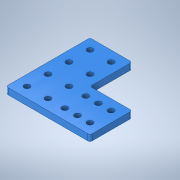
# Autodesk Inventor part: 90deg_4040Bracket
Saved by Autodesk Inventor 2021 (Build 250183000, 183)
## iProperties
Created: 2021-02-03
Part Number: 90deg_4040Bracket
Material: Generic
Document SubType Name: Modeling
Designer: Jorian Brusind
Density: 1 g/cm^3
Appearance: Cyan
Author: Jorian Brusind
Autodesk Inventor part; units mm, degrees
ref_plane "YZ Plane" through (0, 0, 0) normal (1, 0, 0) x (0, 1, 0)
ref_plane "XZ Plane" through (0, 0, 0) normal (0, 1, 0) x (-1, 0, 0)
ref_plane "XY Plane" through (0, 0, 0) normal (0, 0, 1) x (1, 0, 0)
sketch "Sketch1" plane through (0, 0, 0) normal (0, 1, 0) x (-1, 0, 0)
  line L0 (0, 0) -> (40, 0)
  line L1 (40, 0) -> (40, -40)
  line L2 (40, -40) -> (0, -40)
  line L3 (0, -40) -> (0, 0)
  line L4 (40, 0) -> (80, 0)
  line L5 (80, 0) -> (80, -80)
  line L6 (80, -80) -> (40, -80)
  line L7 (40, -80) -> (40, 0)
  dimension "d0" = 40
  dimension "d1" = 40
  dimension "d2" = 40
  dimension "d3" = 80
  constraints: 16 end point, 4 parallel, 2 horizontal, 2 perpendicular
  measures "d0" distance of L1.end L2.end
  measures "d1" distance of L0.end L1.end
  measures "d2" distance of L5.end L6.end
  measures "d3" distance of L4.end L5.end
extrude "Extrusion1" add sketch "Sketch1" along normal blind 6
sketch "Sketch2" plane through (0, 6, 0) normal (0, 1, 0) x (1, 0, 0)
  line L0 (0, 0) -> (0, 40) projected
  line L1 (0, 0) -> (0, 10)
  line L2 (0, 40) -> (0, 30)
  circle A0 centre (-10, 10) radius 2.75
  line L3 (-80, 0) -> (0, 0) projected
  circle A1 centre (-22, 10) radius 2.75
  circle A2 centre (-34, 10) radius 2.75
  circle A3 centre (-10, 30) radius 2.75
  circle A4 centre (-22, 30) radius 2.75
  circle A5 centre (-34, 30) radius 2.75
  circle A6 centre (-70, 70) radius 2.75
  line L4 (-80, 80) -> (-80, 0) projected
  line L5 (-40, 80) -> (-80, 80) projected
  circle A7 centre (-70, 50) radius 2.75
  circle A8 centre (-70, 30) radius 2.75
  circle A9 centre (-70, 10) radius 2.75
  circle A10 centre (-50, 70) radius 2.75
  circle A11 centre (-50, 50) radius 2.75
  circle A12 centre (-50, 30) radius 2.75
  circle A13 centre (-50, 10) radius 2.75
  dimension "d6" = 10
  dimension "d7" = 10
  dimension "d8" = 5.5
  dimension "d9" = 10
  dimension "d10" = 10
  dimension "d13" = 12
  dimension "d16" = 20
  dimension "d19" = 5.5
  dimension "d20" = 10
  dimension "d21" = 10
  dimension "d24" = 20
  dimension "d27" = 20
  constraints: 14 centre point, 4 end point, 2 horizontal, 2 point on line, 2 vertical, 24 other
  measures "d6" distance of L0.start L1.end
  measures "d7" distance of L0.end L2.end
  measures "d8" diameter of A0
  measures "d9" distance from line of L3 A0.centre
  measures "d10" distance from line of L0 A0.centre
  measures "d13" distance of A0.centre A1.centre
  measures "d16" distance of A0.centre A3.centre
  measures "d19" diameter of A6
  measures "d20" distance from line of L4 A6.centre
  measures "d21" distance from line of L5 A6.centre
  measures "d24" distance of A6.centre A7.centre
  measures "d27" distance of A6.centre A10.centre
extrude "Extrusion2" cut sketch "Sketch2" against normal up to next
fillet "Fillet1" radius 2 6 edges at (0, 3, 0) (0, 3, -40) (-40, 3, -80) (-80, 3, 0) (-80, 3, -80) (-40, 3, -40)
body "Solid1"
